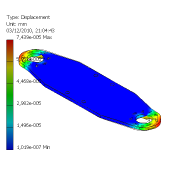
# Autodesk Inventor part: Thigh
Saved by Autodesk Inventor 2011 (Build 150239000, 239)
## iProperties
Created: 2010-11-21
Part Number: Thigh
Document SubType Name: Modeling
Designer: Milton
Density: 2.71 g/cm^3
Mass: 24.4528 g
Surface Area: 84.3059 cm^2
Volume: 9.02318 cm^3
Material: Aluminum-6061
Author: Milton
Autodesk Inventor part; units mm, degrees
ref_plane "YZ Plane" through (0, 0, 0) normal (1, 0, 0) x (0, 1, 0)
ref_plane "XZ Plane" through (0, 0, 0) normal (0, 1, 0) x (-1, 0, 0)
ref_plane "XY Plane" through (0, 0, 0) normal (0, 0, 1) x (1, 0, 0)
sketch "Sketch1" plane through (0, 0, 0) normal (0, 0, 1) x (1, 0, 0)
  line L0 (38.8522, 283.8417) -> (93.8522, 283.8417)
  line L1 (38.8522, 319.8417) -> (93.8522, 319.8417)
  arc A0 (10.8096, 312.4813) -> (10.8096, 291.2021) centre (13.6022, 301.8417) ccw
  line L2 (38.8522, 319.8417) -> (10.8096, 312.4813)
  line L3 (38.8522, 283.8417) -> (10.8096, 291.2021)
  arc A1 (121.8948, 291.2021) -> (121.8948, 312.4813) centre (119.1022, 301.8417) ccw
  line L4 (93.8522, 319.8417) -> (121.8948, 312.4813)
  line L5 (93.8522, 283.8417) -> (121.8948, 291.2021)
  circle A2 centre (13.6022, 301.8417) radius 5
  circle A3 centre (119.1022, 301.8417) radius 5
  circle A4 centre (58.3522, 316.3417) radius 1.5
  circle A5 centre (74.3522, 316.3417) radius 1.5
  circle A6 centre (58.3522, 287.3417) radius 1.5
  circle A7 centre (74.3522, 287.3417) radius 1.5
  dimension "d5" = 36
  dimension "d6" = 105.5
  dimension "d7" = 105.5
  dimension "d8" = 25.25
  dimension "d9" = 25.25
  dimension "d10" = 25.25
  dimension "d11" = 16
  dimension "d12" = 16
  dimension "d13" = 19.5
  dimension "d14" = 19.5
  constraints: 12 end point, 8 centre point, 4 point on circle
  measures "d5" distance between parallel lines of L0 L1
  measures "d6" distance of A0.centre A1.centre
  measures "d7" distance of A3.centre A0.centre
  measures "d8" horizontal distance of L1.start A0.centre
  measures "d9" horizontal distance of L1.end A3.centre
  measures "d10" horizontal distance of L0.end A1.centre
  measures "d11" distance of A6.centre A7.centre
  measures "d12" distance of A5.centre A4.centre
  measures "d13" horizontal distance of L1.start A4.centre
  measures "d14" horizontal distance of L0.start A6.centre
extrude "Extrusion1" add sketch "Sketch1" along normal blind 2.5
sketch "Sketch2" plane through (0, 0, 2.5) normal (0, 0, 1) x (1, 0, 0)
  circle A0 centre (13.6022, 301.8417) radius 5 projected
  circle A1 centre (22.1022, 301.8417) radius 1
  point P0 (0, 0)
  dimension "d15" = 2
  dimension "d16" = 8.5
  constraints: 1 centre point
  measures "d15" diameter of A1
  measures "d16" distance of A1.centre A0.centre
extrude "Extrusion2" cut sketch "Sketch2" against normal through all contours A1
pattern_circular "Circular Pattern1" count 8 over 360 about axis through (13.6022, 301.8417, 0) along (0, 0, 1) of "Extrusion2"
sketch "Sketch3" plane through (0, 0, 2.5) normal (0, 0, 1) x (1, 0, 0)
  circle A0 centre (5.1022, 301.8417) radius 1 projected
  line L0 (93.8522, 319.8417) -> (38.8522, 319.8417) projected
  line L1 (66.3522, 319.8417) -> (66.3522, 283.8417)
  line L2 (38.8522, 283.8417) -> (93.8522, 283.8417) projected
  circle A1 centre (127.6022, 301.8417) radius 1
  point P0 (0, 0)
  constraints: 2 end point, 2 midpoint, 1 centre point, 1 symmetric about line, 1 other
extrude "Extrusion3" cut sketch "Sketch3" against normal through all contours A1
pattern_circular "Circular Pattern2" count 8 over 360 about axis through (119.1022, 301.8417, 0) along (0, 0, 1) of "Extrusion3"
body "Solid1"
